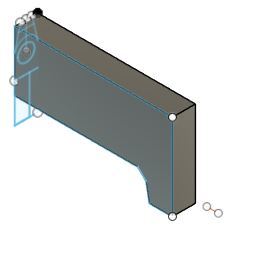
parking_wing_left v2 (Autodesk Fusion 360 design; units mm, degrees)
Autodesk Fusion 360 part; units mm, degrees
sketch "Sketch1" plane through (0, 0, 0) normal (0, 1, 0) x (1, 0, 0)
  line L0 (12, -29) -> (16, -29) construction
  line L1 (0, -50) -> (0, -20)
  line L2 (0, -50) -> (-55, -50)
  line L3 (-55, -50) -> (-55, -29)
  line L4 (-55, -29) -> (-12, -29)
  line L5 (-12, -29) -> (-9.1716, -26.1716)
  line L6 (-9.1716, -26.1716) -> (-8, -20)
  line L7 (0, -20) -> (-8, -20)
  dimension "d3" = 30
  constraint horizontal L0
  constraint symmetric L2.start L1 L1.start
  constraint symmetric L7.start L1 L1.end
  constraint symmetric L0.start L1 L4.end
  measures "d3" distance of L1.start L1.end
extrude "Extrude1" add sketch "Sketch1" along normal blind 8
sketch "Sketch3" plane through (-55, 0, 0) normal (-1, 0, 0) x (0, -1, 0)
  line L0 (0, 29) -> (0, 50)
  line L1 (0, 50) -> (-8, 50)
  line L2 (-8, 50) -> (-8, 29)
  line L3 (-8, 29) -> (0, 29)
  line L4 (-8, 50) -> (-4, 50)
  line L5 (-4, 50) -> (-4, 40)
  line L6 (-6.6394, 47.4424) -> (-1.3606, 47.4424)
  line L7 (0, 42) -> (-2, 50)
  line L8 (-8, 42) -> (-6, 50)
  arc A0 (0, 42) -> (-8, 42) centre (-4, 40.8333) ccw
  circle A1 centre (-4, 40) radius 2.8
  circle A2 centre (-4, 40) radius 3
  line L9 (-2.85, 33.5) -> (-8, 33.5)
  line L10 (0, 33.5) -> (-2.85, 33.5)
  line L11 (0, 20) -> (-2.85, 20)
  line L12 (-2.85, 20) -> (-8, 20)
  line L13 (-8, 33.5) -> (-5.15, 33.5)
  line L14 (-5.15, 33.5) -> (-5.15, 20)
  line L15 (-5.15, 33.5) -> (0, 33.5)
  line L16 (0, 33.5) -> (0, 20)
  line L17 (0, 20) -> (-5.15, 20)
  line L18 (-5.15, 20) -> (-5.15, 33.5)
  dimension "d9" = 5.6
  dimension "d10" = 6
  dimension "d11" = 10
  dimension "d12" = 13.5
  dimension "d13" = 2.85
  dimension "d15" = 2.85
  constraint coincident L1.end L2.start
  constraint midpoint L1 L4.end
  constraint coincident L5.end A1.centre
  constraint concentric A1 A2
  constraint symmetric L7.start L8.start L5
  constraint symmetric L7.end L8.end L5
  constraint coincident L6.start L8
  constraint coincident L6.end L7
  constraint perpendicular L5 L6
  constraint horizontal L11
  constraint horizontal L12
  constraint perpendicular L2 L13
  constraint coincident L12 L14.end
  constraint perpendicular L12 L14
  constraint horizontal L15
  constraint vertical L16
  constraint horizontal L17
  constraint vertical L18
  measures "d9" diameter of A1
  measures "d10" diameter of A2
  measures "d11" distance of L5.end L4.end
  measures "d12" distance of L11.start L10.start
  measures "d13" distance of L10.start L9.start
  measures "d15" distance of L9.end L13.end
extrude "Extrude2" [suppressed]
extrude "Extrude3" [suppressed]
extrude "Extrude4" [suppressed]
fillet "Fillet1" [suppressed]
fillet "Fillet2" [suppressed]
sketch "Sketch4" plane through (0, 8, 0) normal (0, 1, 0) x (-1, 0, 0)
  line L0 (55, 42) -> (0, 42)
  line L1 (0, 42) -> (0, 20)
  line L2 (0, 20) -> (8, 20)
  line L3 (8, 20) -> (9.1716, 26.1716)
  line L4 (9.1716, 26.1716) -> (12, 29)
  line L5 (12, 29) -> (55, 29)
  line L6 (55, 29) -> (55, 40)
  line L7 (55, 40) -> (55, 42)
  circle A0 centre (4, 24) radius 3
  circle A1 centre (4, 37.5) radius 3
  circle A2 centre (4, 37.5) radius 1.5
  line L8 (4, 24) -> (4, 37.5)
  line L9 (4, 20) -> (4, 24)
  circle A3 centre (4, 24) radius 1.5
  line L10 (8, 20) -> (4, 20)
  dimension "d26" = 4
  dimension "d27" = 6
  dimension "d28" = 3
  dimension "d29" = 13.5
  dimension "d30" = 6
  dimension "d31" = 3
  constraint perpendicular L9 L10
  constraint coincident A0.centre L8.start
  constraint concentric A0 A3
  constraint parallel L8 L9
  constraint coincident A1.centre A2.centre
  constraint concentric A1 A2
  measures "d26" distance of L9.start A0.centre
  measures "d27" diameter of A0
  measures "d28" diameter of A3
  measures "d29" distance of A1.centre A0.centre
  measures "d30" diameter of A1
  measures "d31" diameter of A2
extrude "Extrude5" [suppressed]
extrude "Extrude6" [suppressed]
extrude "Extrude7" [suppressed]
fillet "Fillet3" [suppressed]
fillet "Fillet4" [suppressed]
